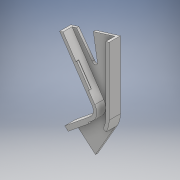
# Autodesk Inventor part: flexible_leg_CS-3_V5_Armor
Saved by Autodesk Inventor 2017 (Build 210142000, 142)
## iProperties
Created: 2017-07-31
Part Number: flexible_leg_CS-3_V5_Armor
Material: Generic
Document SubType Name: Modeling
Designer: Andi
Density: 1 g/cm^3
Appearance: Default
Author: Andi
Autodesk Inventor part; units mm, degrees
ref_plane "YZ Plane" through (0, 0, 0) normal (1, 0, 0) x (0, 1, 0)
ref_plane "XZ Plane" through (0, 0, 0) normal (0, 1, 0) x (-1, 0, 0)
ref_plane "XY Plane" through (0, 0, 0) normal (0, 0, 1) x (1, 0, 0)
sketch "Sketch1" plane through (0, 0, 0) normal (0, 1, 0) x (-1, 0, 0)
  line L0 (0, 0) -> (0, 38)
  arc A0 (23.7631, 30.7092) -> (0, 38) centre (13, 38) ccw
  line L1 (0, 38) -> (13, 38)
  arc A1 (0, 0) -> (1.2058, -4.5) centre (9, 0) ccw
  line L2 (0, 0) -> (9, 0)
  line L3 (0, 0) -> (4, 0)
  arc A2 (4, 0) -> (5.8452, -3.8791) centre (9, 0) ccw
  arc A3 (4.8604, 2.8042) -> (4, 0) centre (9, 0) ccw
  line L4 (23.7631, 30.7092) -> (4.8604, 2.8042)
  line L5 (1.2058, -4.5) -> (12.7058, -24.4186)
  line L6 (12.7058, -24.4186) -> (17.9019, -21.4186)
  arc A4 (12.7058, -24.4186) -> (21.6877, -16.7637) centre (17.9019, -21.4186) ccw
  line L7 (5.8452, -3.8791) -> (21.6877, -16.7637)
  line L8 (20.5183, 23.2445) -> (6.1023, 1.9629)
  line L9 (18.2279, -12.0164) -> (6.7916, -2.7153)
  arc A5 (6.1023, 1.9629) -> (6.7916, -2.7153) centre (9, 0) ccw
  line L10 (-1.5, 30) -> (-1.5, 0)
  line L11 (8.567, -20.25) -> (-0.0933, -5.25)
  arc A6 (-1.5, 0) -> (-0.0933, -5.25) centre (9, 0) ccw
  line L12 (18.2279, -12.0164) -> (8.567, -20.25)
  line L13 (20.5183, 23.2445) -> (-1.5, 30)
  line L14 (4.8604, 2.8042) -> (19.0183, 23.7047)
  line L15 (0, 29.5398) -> (0, 0)
  line L16 (5.8452, -3.8791) -> (17.0671, -13.0058)
  line L17 (9.7278, -19.2607) -> (1.2058, -4.5)
  line L18 (1.2058, -4.5) -> (-0.0933, -5.25)
  dimension "d0" = 38
  dimension "d1" = 13
  dimension "d2" = 9
  dimension "d3" = 5
  dimension "d4" = 30
  dimension "d5" = 23
  dimension "d6" = 6
  dimension "d7" = 4
  dimension "d13" = 1.5
  dimension "d14" = 1.5
  dimension "d15" = 79.561
  dimension "d16" = 79.561
  dimension "d17" = 72.943
  dimension "d18" = 72.943
  dimension "d19" = 30
  dimension "d20" = 15
  constraints: 38 end point, 14 point on circle, 11 tangent, 8 point on line, 7 centre point, 4 parallel, 3 coincident, 2 collinear, 2 concentric, 2 horizontal, 2 perpendicular, 1 vertical
  measures "d0" distance of L0.start L0.end
  measures "d1" distance of L4.start L1.end
  measures "d2" distance of L2.end L0.start
  measures "d3" distance of L3.end L2.end
  measures "d5" distance of L5.start L5.end
  measures "d6" distance of L5.end L6.end
  measures "d7" distance of L3.end L0.start
  measures "d13" distance between parallel lines of L4 L8
  measures "d14" distance between parallel lines of L10 L0
  measures "d15" angle of L12 L9
  measures "d16" angle of L11 L12
  measures "d17" angle of L8 L13
  measures "d18" angle of L10 L13
  measures "d19" vertical distance of L10.start point (0, 0)
  measures "d20" vertical distance of L11.start L11.end
extrude "Extrusion1" add sketch "Sketch1" along normal blind 1 contours A1 L18 A6 L10 L13 L0 | L2 A2 L7 L12 L5 A1 | L0 L13 L4 A3 L2 | L5 L12 L11 L18 | A3 L4 L13 L8 A5 L2 | L2 A5 L9 L12 L7 A2
extrude "Extrusion2" add sketch "Sketch1" against normal blind 4 contours A1 L18 A6 L10 L13 L0 | A3 L4 L13 L8 A5 L2 | L2 A5 L9 L12 L7 A2
sketch "Sketch2" plane through (-5.8452, -4, -3.8791) normal (0.6309641, 0, -0.775812) x (-0.775812, 0, -0.6309641)
  line L0 (14.4647, 0) -> (0, 0) projected
  line L1 (14.4647, 0) -> (2.4647, 0)
  line L2 (2.4647, 1) -> (14.4647, 1)
  line L3 (14.4647, 4) -> (14.4647, 0) projected
  line L4 (14.4647, 0) -> (14.4647, 1)
  line L5 (2.4647, 1) -> (2.4647, 0)
  point P0 (-6.9823, 4)
  dimension "d28" = 12
  constraints: 8 end point, 2 parallel, 2 point on line, 1 collinear
  measures "d28" distance of L2.start L2.end
extrude "Extrusion4" add sketch "Sketch2" along normal blind 0.5
sketch "Sketch3" plane through (-19.0183, -4, 23.7047) normal (0.8279279, 0, 0.5608345) x (0.5608345, 0, -0.8279279)
  line L0 (25.2444, 0) -> (0, 0) projected
  line L1 (20.2444, 0) -> (10.2444, 0)
  line L2 (10.2444, 1) -> (20.2444, 1)
  line L3 (20.2444, 1) -> (20.2444, 0)
  line L4 (10.2444, 1) -> (10.2444, 0)
  point P0 (30.2919, 4)
  dimension "d31" = 10
  dimension "d32" = 5
  dimension "d33" = 1
  constraints: 8 end point, 2 point on line, 1 horizontal, 1 parallel, 1 perpendicular
  measures "d31" distance of L2.start L2.end
  measures "d32" distance from line of L3 L0.start
  measures "d33" distance of L2.start L1.end
extrude "Extrusion5" add sketch "Sketch3" along normal blind 0.5
chamfer "Chamfer1" distance 0.25 angle 45 4 edges at (-12.4122, -3, -9.22) (-10.4687, -3, 11.0835) (-10.0547, -3, 11.3639) (-12.0967, -3, -9.6079)
sketch "Sketch4" plane through (0, 1, 0) normal (0, 1, 0) x (1, 0, 0)
  line L0 (-20.5183, -23.2445) -> (1.5, -30) projected
  line L1 (-17, -24.3239) -> (-10.0702, -14.9785)
  line L2 (-7.7185, -15.7) -> (-9.5091, -26.6222)
  arc A0 (-7.7185, -15.7) -> (-10.0702, -14.9785) centre (-8.9434, -15.4992) ccw
  point P0 (0, 0)
  constraints: 4 end point, 2 point on circle, 1 centre point, 1 midpoint, 1 point on line, 1 tangent
extrude "Extrusion6" cut sketch "Sketch4" against normal blind 10
equation "\"d0\" = d8"
equation "\"d3\" = d2 - d7"
equation "\"d4\" = d9"
equation "\"d5\" = d10"
equation "\"d6\" = d11"
equation "\"d7\" = d12"
equation "\"d15\" = d16"
equation "\"d17\" = d18"
equation "\"d8\" = 38"
equation "\"d9\" = 30deg"
equation "\"d10\" = 23"
equation "\"d11\" = 6"
equation "\"d12\" = 4"
body "Solid1"
